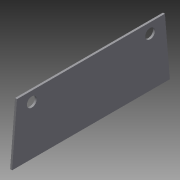
# Autodesk Inventor part: mountPiece
Saved by Autodesk Inventor 2015 SP1 (Build 190203100, 203)
## iProperties
Created: 2015-02-16
Part Number: mountPiece
Material: Generic
Document SubType Name: Modeling
Designer: 55221
Density: 1 g/cm^3
Appearance: Default
Author: 55221
Autodesk Inventor part; units mm, degrees
ref_plane "YZ Plane" through (0, 0, 0) normal (1, 0, 0) x (0, 1, 0)
ref_plane "XZ Plane" through (0, 0, 0) normal (0, 1, 0) x (-1, 0, 0)
ref_plane "XY Plane" through (0, 0, 0) normal (0, 0, 1) x (1, 0, 0)
sketch "Sketch1" plane through (0, 0, 0) normal (1, 0, 0) x (0, 1, 0)
  line L0 (50.8, 190.5) -> (0, 190.5)
  line L1 (0, 190.5) -> (0, 0)
  line L2 (0, 0) -> (50.8, 0)
  line L3 (50.8, 0) -> (50.8, 190.5)
  line L4 (0, 196.85) -> (50.8, 190.5)
  line L5 (0, 196.85) -> (0, 190.5)
  line L6 (0, 0) -> (50.8, 0)
  line L7 (0, 0) -> (0, 0)
  line L8 (50.8, 0) -> (0, 0)
  line L9 (0, 0) -> (0, 0)
  line L10 (0, -6.35) -> (50.8, 0)
  line L11 (0, -6.35) -> (0, 0)
  line L12 (0, 0) -> (76.2, 0)
  line L13 (76.2, 0) -> (76.2, 190.5)
  line L14 (76.2, 190.5) -> (0, 196.85)
  line L15 (76.2, 0) -> (0, -6.35)
  dimension "d0" = 76.2
  constraints: 32 end point, 4 perpendicular, 2 horizontal, 2 parallel, 1 collinear, 1 point on line, 1 vertical
  measures "d0" distance of L8.end L12.end
extrude "Extrusion1" add sketch "Sketch1" along normal blind 2.54
sketch "Sketch2" plane through (2.54, 0, 0) normal (1, 0, 0) x (0, 0, -1)
  circle A0 centre (-19.05, 63.5) radius 6.35
  circle A1 centre (-171.45, 63.5) radius 6.35
  point P0 (0, 0)
  dimension "d3" = 12.7
  dimension "d4" = 12.7
  constraints: 2 centre point
  measures "d3" diameter of A0
  measures "d4" diameter of A1
extrude "Extrusion2" cut sketch "Sketch2" against normal blind 2.54
body "Solid1"
